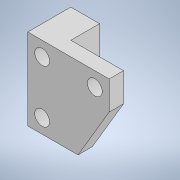
# Autodesk Inventor part: Support Vis rotation
Saved by Autodesk Inventor 2022 (Build 260153000, 153)
## iProperties
Created: 2022-05-03
Part Number: Support Vis rotation
Material: Générique
Document SubType Name: Modeling
Designer: victo
Density: 1 g/cm^3
Appearance: Par défaut
Author: victo
Autodesk Inventor part; units mm, degrees
ref_plane "YZ Plane" through (0, 0, 0) normal (1, 0, 0) x (0, 1, 0)
ref_plane "XZ Plane" through (0, 0, 0) normal (0, 1, 0) x (-1, 0, 0)
ref_plane "XY Plane" through (0, 0, 0) normal (0, 0, 1) x (1, 0, 0)
sketch "Esquisse1" plane through (0, 0, 0) normal (0, 0, 1) x (1, 0, 0)
  line L0 (5.5, -5.5) -> (-5.5, -5.5) construction
  line L1 (-5.5, -5.5) -> (-5.5, 5.5) construction
  line L2 (-5.5, 5.5) -> (5.5, 5.5) construction
  line L3 (5.5, 5.5) -> (5.5, -5.5) construction
  line L4 (5.5, -5.5) -> (-5.5, 5.5) construction
  line L5 (-5.5, -5.5) -> (5.5, 5.5) construction
  circle A0 centre (-5.5, 5.5) radius 1.55
  circle A1 centre (-5.5, -5.5) radius 1.55
  circle A2 centre (5.5, 5.5) radius 1.55
  line L6 (-2.5, -8.5) -> (-8.5, -8.5)
  line L7 (-8.5, -8.5) -> (-8.5, 8.5)
  line L8 (-8.5, 8.5) -> (-2.5, 8.5)
  line L9 (-2.5, 8.5) -> (-2.5, -8.5)
  line L10 (-2.5, -8.5) -> (-8.5, 8.5) construction
  line L11 (-8.5, -8.5) -> (-2.5, 8.5) construction
  line L12 (8.5, 2.5) -> (-8.5, 2.5)
  line L13 (-8.5, 2.5) -> (-8.5, 8.5)
  line L14 (-8.5, 8.5) -> (8.5, 8.5)
  line L15 (8.5, 8.5) -> (8.5, 2.5)
  line L16 (8.5, 2.5) -> (-8.5, 8.5) construction
  line L17 (-8.5, 2.5) -> (8.5, 8.5) construction
  line L18 (-2.5, -8.5) -> (2, -8.5)
  line L19 (8.5, 2.5) -> (2, -8.5)
  point P0 (0, 0)
  point P1 (-5.5, 0)
  point P2 (0, 5.5)
  point P3 (-2.5, 8.5)
  point P4 (-2.5, 2.5)
  dimension "d0" = 11
  dimension "d1" = 3.1
  dimension "d2" = 6
  dimension "d8" = 4.5
  constraints: 40 end point, 8 midpoint, 6 parallel, 5 perpendicular, 3 centre point, 3 coincident, 3 horizontal, 2 equal radius, 1 point on line
  measures "d0" distance of L1.end L2.end
  measures "d1" diameter of A2
  measures "d2" distance between parallel lines of L7 L9
  measures "d8" distance of L6.start L18.end
extrude "Extrusion1" add sketch "Esquisse1" against normal blind 6 contours L6 L7 L12 L9 | L12 L7 L8 L9
extrude "Extrusion2" add sketch "Esquisse1" along normal blind 3
